Autodesk Fusion 360 part; units mm, degrees
(part 7 of 7)
sketch "Sketch15" plane through (0, 1.3065, 0) normal (0, -1, 0) x (1, 0, 0)
  line L0 (25.9951, 21.8729) -> (14.6351, 33.3929)
  line L1 (14.6351, 33.3929) -> (12.6351, 33.3929)
  line L2 (12.6351, 33.3929) -> (12.6351, 20.3929)
  line L3 (12.6351, 20.3929) -> (22.6351, 20.3929)
  line L4 (22.6351, 20.3929) -> (24.6351, 18.3929)
  line L5 (24.6351, 18.3929) -> (24.6351, 3.3929)
  line L6 (24.6351, 3.3929) -> (-19.7086, 3.3929)
  line L7 (-19.7086, 3.3929) -> (-19.7086, -0.6071)
  line L8 (-19.7086, -0.6071) -> (29.6351, -0.6071)
  line L9 (29.6351, -0.6071) -> (29.6351, 9.3929)
  line L10 (29.6351, 9.3929) -> (25.9951, 21.8729)
  line L11 (24.6351, 3.3929) -> (24.6351, -0.6071)
  constraint coincident L5.end L6.start
  constraint coincident L8 L11.end
  constraint perpendicular L8 L11
extrude "Extrude17" add sketch "Sketch15" along normal blind 1 contours L6 L7 L8 L11 bodies 20
extrude "Extrude18" add 1 faces at (24.6351, 0.9732, 2.0595) along direction (1, 0, 0) blind 5 on bodies 20 bodies 20
sketch "Sketch16" plane through (0, 14.3065, 0) normal (0, 1, 0) x (-1, 0, 0)
  line L0 (-14.6351, 33.3929) -> (-25.9951, 21.8729)
  line L1 (-25.9951, 21.8729) -> (-29.6351, 9.3929)
  line L2 (-29.6351, 9.3929) -> (-29.6351, -0.6071)
  line L3 (-29.6351, -0.6071) -> (-24.6351, -0.6071)
  line L4 (-24.6351, -0.6071) -> (-24.6351, 18.3929)
  line L5 (-24.6351, 18.3929) -> (-22.6351, 20.3929)
  line L6 (-22.6351, 20.3929) -> (-12.6351, 20.3929)
  line L7 (-12.6351, 20.3929) -> (-12.6351, 33.3929)
  line L8 (-12.6351, 33.3929) -> (-14.6351, 33.3929)
  line L9 (-24.6351, 18.3929) -> (-27.0101, 18.3929)
  constraint coincident L4.end L5.start
  constraint coincident L1 L9.end
  constraint perpendicular L4 L9
extrude "Extrude19" add sketch "Sketch16" along normal blind 4.5 contours L0 L1 L5 L6 L7 L8 L9 bodies 20
chamfer "Chamfer14" distance 5 angle 45 1 edges at (12.6351, 10.0565, 20.3929) on bodies 20
chamfer "Chamfer15" distance 5 angle 45 1 edges at (17.6351, 10.0565, 20.3929) on bodies 20
sketch "Sketch17" plane through (24.6351, 0, 0) normal (-1, 0, 0) x (0, -1, 0)
  line L0 (-1.3065, 18.3929) -> (-14.3065, 18.3929)
  line L1 (-14.3065, 18.3929) -> (-14.3065, -0.6071)
  line L2 (-14.3065, -0.6071) -> (-3.1065, -0.6071)
  line L3 (-3.1065, -0.6071) -> (-3.1065, 3.3929)
  line L4 (-3.1065, 3.3929) -> (-1.3065, 3.3929)
  line L5 (-1.3065, 3.3929) -> (-1.3065, 18.3929)
  line L6 (-11.8065, 15) -> (-3.8065, 15)
  line L7 (-3.8065, 15) -> (-3.8065, 5)
  line L8 (-3.8065, 5) -> (-11.8065, 5)
  line L9 (-11.8065, 5) -> (-11.8065, 15)
  dimension "d78" = 2.5
  constraint horizontal L6
  constraint vertical L7
  constraint horizontal L8
  constraint vertical L9
  measures "d78" distance of L1 L6.start
extrude "Extrude21" cut sketch "Sketch17" against normal blind 10 contours L6 L7 L8 L9 bodies 20
chamfer "Chamfer16" distance 5 angle 45 1 edges at (27.1351, 14.3065, -0.6071) on bodies 20
sketch "Sketch18" plane through (0, 18.8065, 0) normal (0, 1, 0) x (-1, 0, 0)
  line L0 (-22.6351, 20.3929) -> (-14.0996, 23.9284)
  line L1 (-14.0996, 23.9284) -> (-12.6351, 25.3929)
  line L2 (-12.6351, 25.3929) -> (-12.6351, 33.3929)
  line L3 (-12.6351, 33.3929) -> (-14.6351, 33.3929)
  line L4 (-14.6351, 33.3929) -> (-25.9951, 21.8729)
  line L5 (-25.9951, 21.8729) -> (-27.0101, 18.3929)
  line L6 (-27.0101, 18.3929) -> (-24.6351, 18.3929)
  line L7 (-24.6351, 18.3929) -> (-22.6351, 20.3929)
  line L8 (-25.6768, 19.3929) -> (-25.0494, 19.3929)
  line L9 (-25.0494, 19.3929) -> (-23.2016, 21.2406)
  line L10 (-23.2016, 21.2406) -> (-14.6661, 24.7762)
  line L11 (-14.6661, 24.7762) -> (-13.6351, 25.8071)
  line L12 (-13.6351, 25.8071) -> (-13.6351, 32.3929)
  line L13 (-13.6351, 32.3929) -> (-14.2168, 32.3929)
  line L14 (-14.2168, 32.3929) -> (-25.1058, 21.3505)
  line L15 (-25.1058, 21.3505) -> (-25.6768, 19.3929)
  dimension "d82" = -1
extrude "Extrude22" cut sketch "Sketch18" against normal blind 25 contours L8 L9 L10 L11 L12 L13 L14 L15 bodies 20
sketch "Sketch19" plane through (24.1147, 0, 23.7798) normal (0.712034, 0, 0.702145) x (0, 1, 0)
  line L0 (1.3065, 13.5009) -> (1.3065, -2.6781)
  line L1 (1.3065, -2.6781) -> (18.8065, -2.6781)
  line L2 (18.8065, -2.6781) -> (18.8065, 13.5009)
  line L3 (18.8065, 13.5009) -> (1.3065, 13.5009)
  line L4 (3, 12) -> (17, 12)
  line L5 (17, 12) -> (17, -1)
  line L6 (17, -1) -> (3, -1)
  line L7 (3, -1) -> (3, 12)
  constraint perpendicular L4 L5
  constraint parallel L4 L6
  constraint parallel L5 L7
  constraint parallel L3 L4
extrude "Extrude23" cut sketch "Sketch19" against normal blind 1 contours L4 L5 L6 L7 bodies 20
sketch "Sketch20" plane through (10.5248, 0, 25.4091) normal (-0.382683, 0, -0.92388) x (0, -1, 0)
  line L0 (-1.3065, -13.1081) -> (-1.3065, -3.8693)
  line L1 (-1.3065, -3.8693) -> (-18.8065, -3.8693)
  line L2 (-18.8065, -3.8693) -> (-18.8065, -13.1081)
  line L3 (-18.8065, -13.1081) -> (-1.3065, -13.1081)
  line L4 (-18, -5) -> (-18, -12)
  line L5 (-18, -12) -> (-2, -12)
  line L6 (-2, -12) -> (-2, -5)
  line L7 (-2, -5) -> (-18, -5)
  constraint perpendicular L4 L5
  constraint parallel L4 L6
  constraint parallel L5 L7
  constraint parallel L2 L4
extrude "Extrude24" cut sketch "Sketch20" against normal blind 1 contours L4 L5 L6 L7 bodies 20
sketch "Sketch21" plane through (29.8365, 0, 8.7023) normal (0.96, 0, 0.28) x (0, 1, 0)
  line L0 (3.8065, 0.7193) -> (3.8065, 6.5601)
  line L1 (3.8065, 6.5601) -> (11.8065, 6.5601)
  line L2 (11.8065, 6.5601) -> (11.8065, 0.7193)
  line L3 (11.8065, 0.7193) -> (14.3065, 0.7193)
  line L4 (14.3065, 0.7193) -> (14.3065, 10.0943)
  line L5 (14.3065, 10.0943) -> (18.8065, 10.0943)
  line L6 (18.8065, 10.0943) -> (18.8065, 13.7193)
  line L7 (18.8065, 13.7193) -> (1.3065, 13.7193)
  line L8 (1.3065, 13.7193) -> (1.3065, 0.7193)
  line L9 (1.3065, 0.7193) -> (3.8065, 0.7193)
  line L10 (11.8065, 6.5601) -> (3.8065, 6.5601)
  line L11 (3.8065, 6.5601) -> (3.8065, 12.0595)
  line L12 (3.8065, 12.0595) -> (11.8065, 12.0595)
  line L13 (11.8065, 12.0595) -> (11.8065, 6.5601)
  constraint perpendicular L10 L11
  constraint parallel L10 L12
  constraint parallel L11 L13
  constraint coincident L0.end L1.start
  constraint perpendicular L0 L10
  constraint coincident L1.end L2.start
extrude "Extrude25" cut sketch "Sketch21" against normal blind 20 contours L1 L10 L11 L12 L13 bodies 20
chamfer "Chamfer17" distance 1 angle 45 1 edges at (27.0101, 16.5565, 18.3929) on bodies 20
hidden bodies 1 2
equation "d23 = ( ( 12.8 * PI ) / 16 ) * 1 mm"
named bodies: "Spur Gear (16 teeth)"
